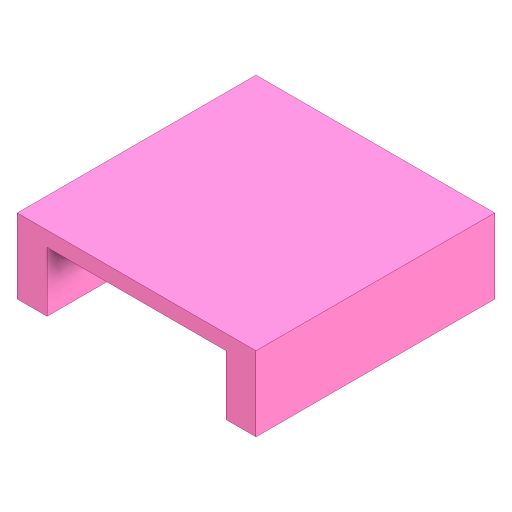
# Autodesk Inventor part: bridge_rect_final
Saved by Autodesk Inventor 2024 (Build 280153000, 153)
## iProperties
Created: 2023-08-28
Part Number: bridge_rect_final
Material: 一般
Document SubType Name: Modeling
Designer: admin
Density: 1 g/cm^3
Appearance: 預設
Author: admin
Autodesk Inventor part; units mm, degrees
ref_plane "YZ Plane" through (0, 0, 0) normal (1, 0, 0) x (0, 1, 0)
ref_plane "XZ Plane" through (0, 0, 0) normal (0, 1, 0) x (-1, 0, 0)
ref_plane "XY Plane" through (0, 0, 0) normal (0, 0, 1) x (1, 0, 0)
sketch "草圖2" plane through (0, 0, 0) normal (0, 0, 1) x (1, 0, 0)
  line L0 (0, 55) -> (0, 0)
  line L1 (0, 0) -> (22, 0)
  line L2 (22, 0) -> (22, 44)
  line L3 (22, 44) -> (154, 44)
  line L4 (154, 44) -> (154, 0)
  line L5 (154, 0) -> (176, 0)
  line L6 (176, 0) -> (176, 55)
  line L7 (176, 55) -> (0, 55)
  dimension "d11" = 22
  dimension "d12" = 11
  dimension "d14" = 176
  dimension "d17" = 44
  constraints: 16 end point, 3 vertical, 2 collinear, 2 horizontal, 2 perpendicular, 1 coincident, 1 parallel
  measures "d11" distance of L0.end L1.end
  measures "d12" distance between parallel lines of L3 L7
  measures "d14" distance of L6.end L0.start
  measures "d17" distance between parallel lines of L1 L3
extrude "擠出2" add sketch "草圖2" along normal mid plane 176
equation "\"d11\" = leg_length"
equation "\"d12\" = thickness"
equation "\"d14\" = width"
equation "\"d17\" = height"
equation "\"d15\" = length"
equation "\"width\" = 80 * ratio"
equation "\"height\" = 20 * ratio"
equation "\"length\" = width"
equation "\"leg_length\" = ratio"
equation "\"ratio\" = 2.2"
equation "\"thickness\" = 5 * ratio"
